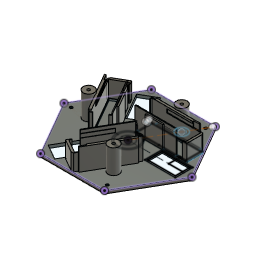
Inside Omniwheels 90D (Autodesk Fusion 360 archive; units mm, degrees)
design "Celluo V2.1 OmniWheels" references "Motor 90 shaft"
Autodesk Fusion 360 part; units mm, degrees
note: some values were not read from the file. Chosen so that the rebuilt part matches the saved one: a direction; a side; which face or edge a step refers to; which sketch regions a step uses.
imported_body "Derived Base Feature3" makes body 1
sketch "Sketch10" plane through (0, 0, 0) normal (0, 1, 0) x (1, 0, 0)
  circle A0 centre (0, 0) radius 46
  line L0 (46, 0) -> (23, 39.8372)
  line L1 (23, 39.8372) -> (-23, 39.8372)
  line L2 (-23, 39.8372) -> (-46, 0)
  line L3 (-46, 0) -> (-23, -39.8372)
  line L4 (-23, -39.8372) -> (23, -39.8372)
  line L5 (23, -39.8372) -> (46, 0)
  line L6 (-21.2679, 36.8372) -> (-42.5359, 0)
  line L7 (-42.5359, 0) -> (-21.2679, -36.8372)
  line L8 (-21.2679, -36.8372) -> (21.2679, -36.8372)
  line L9 (21.2679, -36.8372) -> (42.5359, 0)
  line L10 (42.5359, 0) -> (21.2679, 36.8372)
  line L11 (21.2679, 36.8372) -> (-21.2679, 36.8372)
  line L12 (-22.134, 38.3372) -> (-44.2679, 0)
  line L13 (-44.2679, 0) -> (-22.134, -38.3372)
  line L14 (-22.134, -38.3372) -> (22.134, -38.3372)
  line L15 (22.134, -38.3372) -> (44.2679, 0)
  line L16 (44.2679, 0) -> (22.134, 38.3372)
  line L17 (22.134, 38.3372) -> (-22.134, 38.3372)
  line L18 (-21.9608, 38.0372) -> (-43.9215, 0)
  line L19 (-43.9215, 0) -> (-21.9608, -38.0372)
  line L20 (-21.9608, -38.0372) -> (21.9608, -38.0372)
  line L21 (21.9608, -38.0372) -> (43.9215, 0)
  line L22 (43.9215, 0) -> (21.9608, 38.0372)
  line L23 (21.9608, 38.0372) -> (-21.9608, 38.0372)
  line L24 (0, 0) -> (23, 39.8372) construction
  circle A1 centre (19.5, 33.775) radius 3.5
  circle A2 centre (19.5, 33.775) radius 2.1
  dimension "d727" = 92
  dimension "d729" = -1.5
  dimension "d730" = -1.8
  dimension "d891" = 7
  dimension "d892" = 39
  dimension "d893" = 4.2
  constraint coincident A0.centre L24.start
  constraint coincident A0 L0.start
  constraint coincident L24 A1.centre
  constraint concentric A1 A2
  measures "d727" diameter of A0
  measures "d891" diameter of A1
  measures "d892" distance of A0.centre A1.centre
  measures "d893" diameter of A2
extrude "Extrude1" add sketch "Sketch10" along normal blind 2 separate body contours L6 L7 L8 L9 L10 L11 A1 | L11 A1 | L10 L11 A1 | L10 L11 A1 | L10 A1 | L18 L19 L20 L21 L22 L23 | A2 makes body 2
sketch "Sketch11" plane through (0, 2, 0) normal (0, 1, 0) x (-1, 0, 0)
  circle A0 centre (0, 0) radius 6.9
  circle A1 centre (0, 0) radius 4.1
  line L0 (0, 0) -> (-28, 0) construction
  line L1 (3.783, -17.05) -> (5.0997, -17.05)
  line L2 (0, 0) -> (-21.2679, -36.8372) construction
  circle A2 centre (-13.5, -23.3827) radius 3.75
  circle A3 centre (-13.5, -23.3827) radius 2.1
  circle A4 centre (0, 0) radius 7.9
  line L3 (5.0997, -19.25) -> (5.1031, -19.95)
  line L4 (-21.9608, -38.0372) -> (21.9608, -38.0372)
  line L5 (21.9608, -38.0372) -> (43.9215, 0)
  line L6 (43.9215, 0) -> (21.9608, 38.0372)
  line L7 (21.9608, 38.0372) -> (-21.9608, 38.0372)
  line L8 (-21.9608, 38.0372) -> (-43.9215, 0)
  line L9 (-43.9215, 0) -> (-21.9608, -38.0372)
  line L10 (-28, 0) -> (-28, -8)
  line L11 (-28, -8) -> (-13.5, -8)
  line L12 (-13.5, -8) -> (1.5, -8)
  line L13 (1.5, -8) -> (1.5, -18)
  line L14 (1.5, -18) -> (-31.5, -18)
  line L15 (-31.5, -18) -> (-31.5, -8)
  line L16 (-28, -8) -> (-31.5, -8)
  line L17 (-28, -7.7) -> (-31.8, -7.7)
  line L18 (-31.8, -18.3) -> (-31.8, -7.7)
  line L19 (1.8, -18.3) -> (-31.8, -18.3)
  line L20 (1.8, -7.7) -> (1.8, -18.3)
  line L21 (-13.5, -7.7) -> (1.8, -7.7)
  line L22 (-28, -7.7) -> (-13.5, -7.7)
  line L23 (-28, -7.1) -> (-32.4, -7.1)
  line L24 (-32.4, -18.9) -> (-32.4, -7.1)
  line L25 (2.4, -18.9) -> (-32.4, -18.9)
  line L26 (2.4, -7.1) -> (2.4, -18.9)
  line L27 (-13.5, -7.1) -> (2.4, -7.1)
  line L28 (-28, -7.1) -> (-13.5, -7.1)
  line L29 (-28, 0) -> (-37.5, 0)
  line L30 (-37.5, 0) -> (-37.5, -5)
  line L31 (-37.5, -5) -> (-18.5, -5)
  line L32 (-18.5, -5) -> (-18.5, 5)
  line L33 (-18.5, 5) -> (-37.5, 5)
  line L34 (-37.5, 5) -> (-37.5, 0)
  line L35 (0, -18.9) -> (0, -19.9)
  line L36 (0, -19.9) -> (-30, -19.9)
  line L37 (-30, -19.9) -> (-30, -18.9)
  line L38 (-33.3242, -17.5) -> (-33.3242, -7.1)
  line L39 (-33.3242, -7.1) -> (-32.4, -7.1)
  line L40 (2.4, -9.0599) -> (1.5, -9.0599)
  line L41 (2.4, -17.2552) -> (1.5, -17.2552)
  line L42 (-5.55, -7.1) -> (-5.55, -6.1)
  line L43 (-5.55, -6.1) -> (-26, -6.1)
  line L44 (-26, -6.1) -> (-26, -7.1)
  line L45 (-17.6828, -6.1) -> (-17.6828, -7.1)
  line L46 (-26, -7.1) -> (-26, -8)
  line L47 (-30.2, -7.1) -> (-30.2, -8)
  line L48 (-38.5, 0) -> (-38.5, -6)
  line L49 (-38.5, -6) -> (-17.5, -6)
  line L50 (-17.5, -6) -> (-17.5, 6)
  line L51 (-17.5, 6) -> (-38.5, 6)
  line L52 (-38.5, 6) -> (-38.5, 0)
  line L53 (-32.4, -18.9) -> (-33.3242, -17.5)
  dimension "d733" = 13.8
  dimension "d734" = 8.2
  dimension "d735" = 28
  dimension "d750" = 7.5
  dimension "d751" = 4.2
  dimension "d752" = 27
  dimension "d803" = 1
  dimension "d977" = 8
  dimension "d980" = 14.5
  dimension "d981" = 15
  dimension "d982" = 10
  dimension "d983" = 33
  dimension "d984" = 10
  dimension "d985" = -0.3
  dimension "d986" = -0.9
  dimension "d987" = 9.5
  dimension "d988" = 5
  dimension "d989" = 19
  dimension "d990" = 10
  dimension "d991" = 19
  dimension "d992" = 1
  dimension "d993" = 1
  dimension "d1000" = 1
  constraint coincident A0.centre A1.centre
  constraint concentric A0 A1
  constraint horizontal L0
  constraint coincident L2 A2.centre
  constraint concentric A2 A3
  constraint perpendicular L0 L10
  constraint perpendicular L10 L11
  constraint perpendicular L10 L12
  constraint perpendicular L13 L14
  constraint perpendicular L14 L15
  constraint perpendicular L15 L16
  constraint perpendicular L10 L29
  constraint perpendicular L29 L30
  constraint perpendicular L30 L31
  constraint perpendicular L31 L32
  constraint perpendicular L32 L33
  constraint coincident L25 L35.start
  constraint perpendicular L25 L35
  constraint perpendicular L35 L36
  constraint coincident L25 L37.end
  constraint perpendicular L25 L37
  constraint coincident L24 L23.end
  constraint perpendicular L24 L39
  constraint coincident L26 L40.start
  constraint coincident L13 L40.end
  constraint perpendicular L13 L40
  constraint coincident L26 L41.start
  constraint coincident L13 L41.end
  constraint perpendicular L13 L41
  constraint midpoint L27 L42.start
  constraint perpendicular L27 L42
  constraint perpendicular L42 L43
  constraint coincident L28 L44.end
  constraint perpendicular L28 L44
  constraint coincident L43 L45.start
  constraint coincident L28 L45.end
  constraint perpendicular L28 L45
  constraint coincident L11 L46.end
  constraint perpendicular L11 L46
  constraint midpoint L23 L47.start
  constraint coincident L16 L47.end
  constraint perpendicular L16 L47
  constraint vertical L38
  constraint collinear L23 L39
  measures "d733" diameter of A0
  measures "d734" diameter of A1
  measures "d735" distance of A0.centre L0.end
  measures "d750" diameter of A2
  measures "d751" diameter of A3
  measures "d752" distance of A0.centre A2.centre
  measures "d977" distance of L0.end L10.end
  measures "d980" distance of L10.end L11.end
  measures "d981" distance of L11.end L12.end
  measures "d982" distance of L12.end L13.end
  measures "d983" distance of L13.end L14.end
  measures "d984" distance of L14.end L15.end
  measures "d987" distance of L0.end L29.end
  measures "d988" distance of L29.end L30.end
  measures "d989" distance of L30.end L31.end
  measures "d990" distance of L31.end L32.end
  measures "d991" distance of L32.end L33.end
  measures "d992" distance of L35.start L35.end
  measures "d993" distance of L42.start L42.end
sketch "Sketch14" plane through (0, 2, 0) normal (0, 1, 0) x (-1, 0, 0)
  line L0 (0, 0) -> (-33, -19) construction
  line L1 (-3.5532, -2.0458) -> (-4.5485, -0.317)
  circle A0 centre (0, 0) radius 4.1
  line L2 (-44, 0) -> (-22, -38)
  line L3 (-21.9608, -38.0372) -> (21.9608, -38.0372)
  line L4 (21.9608, -38.0372) -> (43.9215, 0)
  line L5 (43.9215, 0) -> (21.9608, 38.0372)
  line L6 (21.9608, 38.0372) -> (-21.9608, 38.0372)
  line L7 (-21.9608, 38.0372) -> (-43.9215, 0)
  line L8 (-43.9215, 0) -> (-21.9608, -38.0372)
  constraint coincident L0.start A0.centre
  constraint coincident L0 L1.start
  constraint perpendicular L0 L1
  constraint tangent L1 A0
  constraint midpoint L0.end L2
ref_plane "WorkPlane3" through (4.0508, 2, -1.1814) normal (-0.750517, -0.5, 0.432116) x (0.498964, 0, 0.866622)
sketch "Sketch15" plane through (4.0508, 2, -1.1814) normal (-0.750517, -0.5, 0.432116) x (0.498964, 0, 0.866622)
  line L0 (-0.9974, 0) -> (-0.9974, 2)
  line L1 (-0.9974, 0) -> (-2.7974, 0)
  line L2 (-2.7974, 0) -> (-2.7974, 2)
  line L3 (-2.7974, 2) -> (-0.9974, 2)
  line L4 (-2.7974, 0) -> (-2.7974, -2)
  line L5 (-2.7974, -2) -> (-0.9977, -2)
  line L6 (-0.9977, -2) -> (-0.9974, 0)
  line L7 (0.8026, 0) -> (0.8026, 2)
  line L8 (0.8026, 2) -> (-0.9974, 2)
  line L9 (0.8026, 0) -> (0.8026, -2)
  line L10 (0.8026, -2) -> (-0.997, -2)
  line L11 (-0.997, -2) -> (-0.9974, 0)
  line L12 (-3.2974, -2.5) -> (-0.9977, -2.5)
  line L13 (-3.2974, 0) -> (-3.2974, -2.5)
  line L14 (-3.2974, 0) -> (-3.2974, 2.5)
  line L15 (-3.2974, 2.5) -> (-0.9974, 2.5)
  line L16 (1.3026, 2.5) -> (-0.9974, 2.5)
  line L17 (1.3026, 0) -> (1.3026, 2.5)
  line L18 (1.3026, 0) -> (1.3026, -2.5)
  line L19 (1.3026, -2.5) -> (-0.997, -2.5)
  line L20 (-0.997, -2.5) -> (-0.9977, -2.5)
  line L21 (-3.2974, -2) -> (1.3026, -2)
  point P0 (-0.9974, 0)
  dimension "d805" = 2
  dimension "d806" = 1.8
  dimension "d807" = 2
  dimension "d940" = 0.5
  constraint coincident P0 L0.start
  constraint perpendicular L0 L1
  constraint perpendicular L1 L2
  constraint perpendicular L1 L4
  constraint perpendicular L4 L5
  constraint symmetric P0 L0 L1.start
  constraint symmetric L3.end L0 L8.end
  constraint symmetric L0 L1.end L7.start
  constraint symmetric L0 L2.end L7.end
  constraint symmetric L0 L4.end L9.end
  constraint symmetric L0 L5.end L10.end
  constraint parallel L12 L20
  constraint coincident L13 L21.start
  constraint coincident L18 L21.end
  constraint perpendicular L18 L21
  measures "d805" distance of P0 L0.end
  measures "d806" distance of P0 L1.end
  measures "d807" distance of L1.end L4.end
extrude "Extrude9" add sketch "Sketch15" against normal blind 3 contours L0 L1 L2 L3 | L1 L4 L5 L6 L11 L21 | L0 L6 L7 L8 L9 L10 L11 L21 | L2 L3 L4 L7 L8 L9 L13 L14 L15 L16 L17 L18 L21 bodies 2
sketch "Sketch16" plane through (5.6669, 3.7754, -3.2628) normal (0.750517, 0.5, -0.432116) x (-0.498964, 0, -0.866622)
  line L0 (-2.3, -2.05) -> (2.3, -2.05)
  line L1 (0.95, -1.25) -> (-0.95, -1.25)
  line L2 (-0.95, -1.25) -> (-0.95, 1.25)
  line L3 (-0.95, 1.25) -> (0.95, 1.25)
  line L4 (0.95, 1.25) -> (0.95, -1.25)
  line L5 (0.95, -1.25) -> (-0.95, 1.25) construction
  line L6 (-0.95, -1.25) -> (0.95, 1.25) construction
  line L7 (2.3, -2.05) -> (2.3, 2.1821)
  line L8 (2.3, 2.1821) -> (-2.3, 2.1821)
  line L9 (-2.3, 2.1821) -> (-2.3, -2.05)
  dimension "d941" = 1.9
  dimension "d942" = 2.5
  constraint horizontal L1
  constraint perpendicular L1 L2
  constraint parallel L1 L3
  constraint parallel L2 L4
  constraint coincident L5 origin
  constraint coincident L6 origin
  measures "d941" distance of L2.end L3.end
  measures "d942" distance of L1.start L3.end
extrude "Extrude10" cut sketch "Sketch16" against normal blind 8.5 contours L1 L2 L3 L4 bodies 2
sketch "Sketch17" plane through (-0.9455, 1.8897, 0.5444) normal (-0.433311, 0.866025, 0.249482) x (0.498964, 0, 0.866622)
  line L0 (-1.8, 4.5507) -> (1.8, 4.5507)
  line L1 (1.8, 7.5507) -> (-1.8, 7.5507)
  line L2 (-1.8, 7.5507) -> (-1.8, 4.5507)
  line L3 (1.8, 4.5507) -> (1.8, 7.5507)
  line L4 (-1.8, 6.0507) -> (1.8, 6.0507) construction
  line L5 (0, 6.0507) -> (-1.5, 6.0507)
  line L6 (-1.5, 6.0507) -> (-1.5, 5.0507)
  line L7 (-1.5, 5.0507) -> (1.5, 5.0507)
  line L8 (1.5, 5.0507) -> (1.5, 7.0507)
  line L9 (1.5, 7.0507) -> (-1.5, 7.0507)
  line L10 (-1.5, 7.0507) -> (-1.5, 6.0507)
  line L11 (1.0425, 7.0507) -> (1.0425, 7.5803)
  line L12 (0, 6.0507) -> (0, 7.5507) construction
  line L13 (-1.0425, 7.0507) -> (-1.0425, 7.5803)
  line L14 (-1.0425, 7.5803) -> (1.0425, 7.5803)
  line L15 (-2.3, 4.5507) -> (2.3, 4.5507)
  line L16 (2.3, 4.5507) -> (2.3, 7.5507)
  line L17 (2.3, 7.5507) -> (-2.3, 7.5507)
  line L18 (-2.3, 7.5507) -> (-2.3, 4.5507)
  dimension "d814" = 1.5
  dimension "d815" = 1
  dimension "d816" = 3
  dimension "d817" = 2
  constraint midpoint L2 L4.start
  constraint midpoint L3 L4.end
  constraint parallel L4 L5
  constraint perpendicular L5 L6
  constraint perpendicular L6 L7
  constraint perpendicular L7 L8
  constraint horizontal L9
  constraint coincident L9 L11.start
  constraint vertical L11
  constraint midpoint L1 L12.end
  constraint perpendicular L1 L12
  constraint symmetric L11.start L12 L13.start
  constraint symmetric L11.end L12 L13.end
  measures "d814" distance of L5.start L5.end
  measures "d815" distance of L5.end L6.end
  measures "d816" distance of L6.end L7.end
  measures "d817" distance of L7.end L8.end
extrude "Extrude12" cut sketch "Sketch17" against normal blind 3.2 contours L1 L11 L13 L14 L17 | L1 L9 L11 L13 L17 | L6 L7 L8 L9 L10 bodies 2
pattern_circular "C-Pattern4" count 3 over 360 about axis through (0, 1.75, 0) along (0, 1, 0) of "Extrude9", "Extrude10", "Extrude12"
extrude "Extrude8" cut sketch "Sketch11" against normal up to surface (2 mm away) contours A1 bodies 2
extrude "Extrude5" add sketch "Sketch11" along normal blind 16.1 contours A2 L36 | A2 L36 | A4 L21 L26 L27 | A4 L21 L22 L27 L28 L46 | A3 bodies 2
extrude "Extrude6" add sketch "Sketch11" along normal blind 15 contours A2 L25 L35 L36 L37 | L17 L18 L19 L20 L23 L24 L25 L26 L41 L47 | L24 L38 L39 L53 | A4 L20 L21 L26 L40 | A4 L21 L26 L27 | A4 L21 L22 L27 L28 L46 | L27 L28 L42 L43 L45 bodies 2
sketch "Sketch22" plane through (0, 17, 0) normal (0, 1, 0) x (-1, 0, 0)
  line L0 (5.0997, -13) -> (3.883, -13)
  line L1 (5.0997, -11.5) -> (3.883, -11.5)
  line L2 (5.0997, -14.5) -> (3.883, -14.5)
  line L3 (1.7664, -7.7) -> (1.8, -7.7)
  line L4 (1.8, -7.7) -> (1.8, -9.0599)
  line L5 (1.8, -9.0599) -> (2.4, -9.0599)
  line L6 (2.4, -9.0599) -> (2.4, -7.5266)
  line L7 (-17.6828, -7.1) -> (-5.55, -7.1)
  line L8 (-5.55, -7.1) -> (-5.55, -6.1)
  line L9 (-5.55, -6.1) -> (-17.6828, -6.1)
  line L10 (-17.6828, -6.1) -> (-17.6828, -7.1)
  line L11 (-12.1095, -19.9) -> (0, -19.9)
  line L12 (0, -19.9) -> (0, -18.9)
  line L13 (0, -18.9) -> (2.4, -18.9)
  line L14 (2.4, -18.9) -> (2.4, -17.2552)
  line L15 (2.4, -17.2552) -> (1.8, -17.2552)
  line L16 (1.8, -17.2552) -> (1.8, -18.3)
  line L17 (1.8, -18.3) -> (-31.8, -18.3)
  line L18 (-31.8, -18.3) -> (-31.8, -7.7)
  line L19 (-31.8, -7.7) -> (-30.2, -7.7)
  line L20 (-30.2, -7.7) -> (-30.2, -7.1)
  line L21 (-30.2, -7.1) -> (-33.3242, -7.1)
  line L22 (-33.3242, -7.1) -> (-33.3242, -17.5)
  line L23 (-32.4, -18.9) -> (-30, -18.9)
  line L24 (-30, -18.9) -> (-30, -19.9)
  line L25 (-30, -19.9) -> (-14.8905, -19.9)
  arc A0 (1.7664, -7.7) -> (2.4, -7.5266) centre (0, 0) ccw
  arc A1 (-12.1095, -19.9) -> (-14.8905, -19.9) centre (-13.5, -23.3827) ccw
  line L26 (-33.3242, -17.5) -> (-32.4, -18.9)
  dimension "d943" = 1.5
  dimension "d944" = 1.5
  measures "d943" distance of L0 L2
  measures "d944" distance of L0 L1
extrude "Extrude7" add sketch "Sketch11" along normal blind 16.5 contours A2 L36 | A2 L36 | A3 bodies 2
sketch "Sketch19" plane through (33.3242, 0, 0) normal (1, 0, 0) x (0, 0, -1)
  line L0 (18.8186, 13.2) -> (18.8186, 15.7)
  line L1 (7.5, 13.2) -> (7.5, 15.7)
  line L2 (7.5, 15.7) -> (18.8186, 15.7)
  line L3 (18.8186, 13.2) -> (7.5, 13.2)
  line L4 (7.57, 15.63) -> (18.7486, 15.63)
  line L5 (18.7486, 13.27) -> (18.7486, 15.63)
  line L6 (18.7486, 13.27) -> (7.57, 13.27)
  line L7 (7.57, 13.27) -> (7.57, 15.63)
  line L8 (6.35, 2) -> (6.4273, 2)
  line L9 (7.3, 2) -> (9, 2)
  line L10 (7.3, 2) -> (7.3, 17)
  line L11 (7.6, 15.63) -> (7.6, 15.9409)
  line L12 (7.6, 15.9409) -> (18, 15.9409)
  line L13 (18, 15.9409) -> (18, 15.7)
  line L14 (0, 2) -> (38.0372, 2)
  line L15 (7.1, 2) -> (17.5, 2)
  line L16 (17.5, 2) -> (17.5, 17)
  line L17 (17.5, 17) -> (7.1, 17)
  line L18 (7.1, 17) -> (7.1, 2)
  line L19 (19.0186, 2) -> (19.0186, 17)
  line L20 (7.1, 13.2) -> (19.0186, 13.2)
  line L21 (19.0186, 13.2) -> (19.0186, 17)
  line L22 (19.0186, 17) -> (7.1, 17)
  dimension "d824" = 2.5
  dimension "d826" = 2.5
  dimension "d828" = -0.07
  dimension "d995" = 0.2
  dimension "d997" = 11.2
  dimension "d1010" = 0.2
  constraint perpendicular L0 L3
  constraint coincident L4 L11.start
  constraint perpendicular L4 L11
  constraint perpendicular L11 L12
  constraint coincident L2 L13.end
  constraint perpendicular L2 L13
  constraint midpoint L14 L19.start
  constraint perpendicular L14 L19
  constraint coincident L18 L20.start
  constraint coincident L19 L20.end
  constraint perpendicular L19 L20
  constraint coincident L17.end L18.start
  measures "d824" distance of L0.start L0.end
  measures "d826" distance of L1.start L1.end
  measures "d995" distance of L1 L10
  measures "d997" distance of L3 L14
  measures "d1010" distance of L0 L19
extrude "Extrude13" cut sketch "Sketch19" against normal blind 25 contours L0 L2 L3 L4 L5 L6 L16 L20 | L1 L2 L3 L4 L6 L7 L11 L16 L20 | L2 L12 L13 L16 | L4 L5 L6 L16 | L4 L6 L7 L16 | L2 L4 L11 L16 | L2 L11 L12 L16 bodies 2
extrude "Extrude22" cut sketch "Sketch19" against normal up to surface (7.3242 mm away) contours L0 L2 L3 L4 L5 L6 L16 L20 | L0 L2 L12 L13 L16 L19 L20 L21 L22 | L1 L2 L3 L4 L6 L7 L11 L16 L20 | L1 L2 L10 L11 L12 L16 L17 L20 L22 | L10 L17 L18 L20 L22 bodies 2
extrude "Extrude14" add sketch "Sketch19" against normal up to surface (24.9 mm away) separate body contours L4 L5 L6 L16 | L4 L6 L7 L16 makes body 3
hole "Hole1" at (13.5, 18.5, -23.3827) direction (0, -1, 0) diameter 1.85 depth 17.4 tip angle 118 bodies 2
extrude "Extrude19" cut sketch "Sketch11" against normal blind 1.2 contours L11 L12 L13 L14 L15 L16 bodies 2
extrude "Extrude20" cut sketch "Sketch11" against normal up to surface (2 mm away) contours L10 L29 L31 L32 L33 L34 | L10 L29 L30 L31 | L48 L49 L50 L51 L52 bodies 2
pattern_circular "C-Pattern5" count 3 over 360 about axis through (0, 1.75, 0) along (0, 1, 0) of "Extrude5", "Extrude6", "Extrude7", "Extrude13", "Extrude22", "Extrude14", "Hole1", "Extrude19", "Extrude20" makes body 4 makes body 5
extrude "Extrude21" cut sketch "Sketch10" along normal blind 0.4 contours A2 bodies 2
hole "Hole6" at (19.5, 0.4, -33.775) direction (0, 1, 0) diameter 2 depth 8 tip angle 118 countersink diameter 4 countersink angle 90 bodies 2
pattern_circular "C-Pattern6" count 3 over 360 about axis through (0, 1.75, 0) along (0, 1, 0) of "Extrude21", "Hole6"
other "ExternalDerived7"
move_body "Move1" bodies 1 to x (0, 1, 0) y (0, 0, 1) z (1, 0, 0) at (-18, 7, 29)
move_body "Move2" bodies 1 to x (1, 0, 0) y (0, 1, 0) z (0, 0, 1) at (16.5316, 0, -42.0606)
hidden bodies 3 4 5 1
equation "BaseDiameter = 92 mm"
equation "CameraHole = 8.2 mm"
equation "BallDiameter = 16 mm"
equation "PCBHeight = 16.5 mm"
equation "PCBDiamete = 60 mm"
equation "OutterWallThickness = 3 mm"
equation "InnerWallThickness = 1 mm"
equation "Tolerance = 0.2 mm"
equation "MotorLenght = 24.4 mm"
equation "MotorDiameter = 12.1 mm"
equation "MotorWidth = 10.1 mm"
equation "MotorShaft = 10 mm" comment "Shaft and preShaft. Shaft 9.3"
equation "MotorMagnetWidth = 5 mm"
equation "MotorMagnetDiameter = 10 mm"
equation "PilarDistance = 27 mm"
equation "PilarDiameter = 7.5 mm"
equation "ScrewPilarDiameter = ScrewDiameter"
equation "ScrewPilarLength = 8 mm"
equation "MotorShaftDiameter = 3 mm"
equation "ScrewLidDiameter = ScrewDiameter"
equation "ScrewLidDistance = BaseDiameter / 2 - OutterWallThickness - ScrewHead"
equation "TopDiameter = 82 mm"
equation "ModuleHeight = 32 mm" comment "Original 30"
equation "CylinderScrewDiameter = 7 mm"
equation "ScrewHead = 4 mm" comment "for m3 5.5 test okey"
equation "CameraHoleBig = 13.8 mm"
equation "DistanceBallToWall = 1 mm"
equation "BallCaseThickness = 2.3 mm"
equation "BallDistance = 28 mm"
equation "BallMiddlePlane = 4.5 mm" comment "Old 4"
equation "BaseThickness = 2 mm"
equation "BottomLidThickness = 1 mm"
equation "BottomLEDWidth = 2.95 mm"
equation "BottomLEDHeight = 3.15 mm"
equation "MotorHole = 0.5 mm"
equation "BearingDiameter = 3 mm"
equation "MotorCylinderLength = 15.3 mm"
equation "SpacerDiameter = 4 mm"
equation "SpacerHeight = 4 mm"
equation "ScrewBottomLidHeight = 8 mm"
equation "ScrewLidHeight = 8 mm"
equation "PogoDistanceCenter = 27.3 mm"
equation "PogoDiameter = 1.7 mm" comment "Old 1.6"
equation "PogoDistance = 2.54 mm"
equation "MagnetConnectDiameter = 4.85 mm"
equation "MagnetConnectDepth = 1.65 mm - 0.15 mm"
equation "MagnetConnectDistanceCenter = 18 mm"
equation "MechanicalLockDistanceCenter = 12 mm"
equation "MechanicalLockLength = 15 mm"
equation "MechanicalLockWidth = 2 mm"
equation "MechanicalLockDepth = 1.5 mm"
equation "MechanicalLockFillet = 1 mm"
equation "BordersSoftness = 0.1 mm"
equation "BorderRadius = 1.5 mm"
equation "LidBallReduction = 2.5 mm"
equation "TouchBandWidth = 10 mm"
equation "ScrewPreHole = 0.4 mm"
equation "ScrewDiameter = 1.85 mm" comment "M2 = 1.85, M3=2.85"
equation "CameraDiameter = 20 mm"
equation "Game = 0.17 mm"
equation "MotorBaseSupport = 0.5 mm"
equation "d727 = BaseDiameter"
equation "d728 = -OutterWallThickness"
equation "d731 = BaseThickness"
equation "d733 = CameraHoleBig"
equation "d734 = CameraHole"
equation "d735 = BallDistance"
equation "MotorPreShaft = 0.7 mm"
equation "d752 = PilarDistance"
equation "d795 = MotorDiameter + 4 mm"
equation "d799 = PCBHeight"
equation "d834 = ScrewDiameter"
equation "d891 = CylinderScrewDiameter"
equation "d892 = ScrewLidDistance"
equation "d893 = ScrewHead + Tolerance"
equation "d1003 = ScrewPreHole"
equation "d1008 = ScrewHead"
equation "d865 = ScrewPreHole"
equation "d878 = ScrewDiameter"
equation "d880 = ScrewHead"
equation "d883 = ScrewDiameter"
equation "d885 = ScrewHead"
equation "d897 = ScrewDiameter"
equation "d899 = 4.00 mm - 0.5 mm"
equation "d902 = ScrewDiameter"
equation "d904 = 4.00 mm - 0.5 mm"
named bodies: "Base", "MotorLid", "MotorLid (1)", "MotorLid (2)", "Body1"

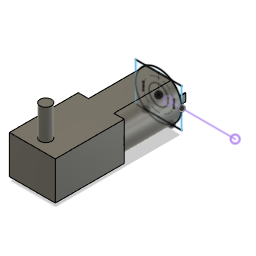
design "Motor 90 shaft"
Autodesk Fusion 360 part; units mm, degrees
sketch "Sketch1" plane through (0, 0, 0) normal (0, 0, 1) x (1, 0, 0)
  circle A0 centre (0, 0) radius 6
  line L0 (0, 0) -> (0, 5) construction
  line L1 (0, 5) -> (3.3166, 5)
  line L2 (0, 5) -> (-3.3166, 5)
  line L3 (20, 0) -> (2.5, 0)
  line L4 (0, -5) -> (3.3166, -5)
  line L5 (0, -5) -> (-3.3166, -5)
  circle A1 centre (0, 0) radius 2.5
  circle A2 centre (0, 0) radius 3.9 construction
  line L6 (-3.9, 0) -> (-3.9, 1)
  line L7 (-3.9, 1) -> (-4.1, 1)
  line L8 (-4.1, 1) -> (-4.1, -1)
  line L9 (-4.1, -1) -> (-3.9, -1)
  line L10 (-3.9, -1) -> (-3.9, 0)
  line L11 (4.1, 1) -> (4.1, -1)
  line L12 (3.9, 0) -> (3.9, 1)
  line L13 (3.9, 1) -> (4.1, 1)
  line L14 (3.9, -1) -> (3.9, 0)
  line L15 (4.1, -1) -> (3.9, -1)
  line L16 (6, 0) -> (6, 5)
  line L17 (6, 5) -> (-6, 5)
  line L18 (-6, 5) -> (-6, -5)
  line L19 (-6, -5) -> (6, -5)
  line L20 (6, -5) -> (6, 0)
  dimension "d1" = 12
  dimension "d2" = 5
  dimension "d5" = 5
  dimension "d8" = 7.8
  dimension "d9" = 1
  dimension "d10" = 0.2
  dimension "d11" = 2
  dimension "d12" = 0.2
  dimension "d15" = 5
  dimension "d16" = 12
  dimension "d17" = 10
  dimension "d18" = 12
  constraint coincident A0.centre L0.start
  constraint vertical L0
  constraint coincident A0 L1.end
  constraint perpendicular L0 L1
  constraint coincident A0 L2.end
  constraint perpendicular L0 L2
  constraint symmetric L0.end L3 L4.start
  constraint symmetric L1.end L3 L4.end
  constraint symmetric L2.end L3 L5.end
  constraint concentric A1 A2
  constraint coincident A2 L6.start
  constraint tangent A2 L6
  constraint vertical L6
  constraint perpendicular L6 L7
  constraint perpendicular L7 L8
  constraint perpendicular L8 L9
  constraint symmetric L0 L6.start L12.start
  constraint symmetric L0 L6.end L12.end
  constraint symmetric L0 L7.end L11.start
  constraint symmetric L0 L8.end L11.end
  constraint symmetric L0 L9.end L14.start
  constraint coincident L3 L16.start
  constraint perpendicular L3 L16
  constraint perpendicular L16 L17
  constraint perpendicular L2 L18
  constraint perpendicular L18 L19
  measures "d1" diameter of A0
  measures "d2" distance of A0.centre L0.end
  measures "d5" diameter of A1
  measures "d8" diameter of A2
  measures "d9" distance of L6.start L6.end
  measures "d10" distance of L6.end L7.end
  measures "d11" distance of L7.end L8.end
  measures "d12" distance of L8.end L9.end
  measures "d15" distance of L16.start L16.end
  measures "d16" distance of L16.end L17.end
  measures "d17" distance of L17.end L18.end
  measures "d18" distance of L18.end L19.end
extrude "Extrude1" add sketch "Sketch1" along normal blind 15 contours A0 L1 L2 L4 L5 L17 L19 | L3 L11 L14 L15 | L3 L11 L12 L13 | A1 | L6 L7 L8 L9 L10
extrude "Extrude2" add sketch "Sketch1" against normal blind 1.7 contours A1
extrude "Extrude3" add sketch "Sketch1" against normal blind 3 contours L3 L11 L14 L15 | L3 L11 L12 L13 | L6 L7 L8 L9 L10
extrude "Extrude4" add sketch "Sketch1" along normal blind 18 from surface at 15 contours A0 L1 L2 L4 L5 L17 L19 | A0 L19 L20 | A0 L16 L17 | A0 L17 L18 | A0 L18 L19 | L3 L11 L14 L15 | L3 L11 L12 L13 | A1 | L6 L7 L8 L9 L10
sketch "Sketch2" plane through (0, 5, 0) normal (0, 1, 0) x (-1, 0, 0)
  line L0 (-15, 0) -> (-15, 5)
  line L1 (-15, 5) -> (-33, 5)
  line L2 (-33, 5) -> (-33, -5)
  line L3 (-33, -5) -> (-15, -5)
  line L4 (-15, -5) -> (-15, 0)
  line L5 (-15, 0) -> (-31, 0) construction
  line L6 (-31, 0) -> (-29.5, 0) construction
  circle A0 centre (-29.5, 0) radius 1.5
  line L7 (-3.3166, 0) -> (3.3166, 0)
  line L8 (3.3166, 0) -> (3.3166, 15)
  line L9 (3.3166, 15) -> (6, 15)
  line L10 (6, 15) -> (6, 33)
  line L11 (6, 33) -> (-6, 33)
  line L12 (-6, 33) -> (-6, 15)
  line L13 (-6, 15) -> (-3.3166, 15)
  line L14 (-3.3166, 15) -> (-3.3166, 0)
  line L15 (3.3166, 15) -> (-3.3166, 15)
  line L16 (0, 15) -> (0, 31) construction
  line L17 (0, 31) -> (0, 29.5) construction
  circle A1 centre (0, 29.5) radius 1.5
  dimension "d22" = 16
  dimension "d23" = 1.5
  dimension "d24" = 3
  dimension "d25" = 16
  dimension "d26" = 1.5
  dimension "d27" = 3
  constraint coincident L0.start L4.end
  constraint perpendicular L0 L5
  constraint parallel L5 L6
  constraint coincident L6.end A0.centre
  constraint coincident L8.end L9.start
  constraint coincident L13.end L14.start
  constraint midpoint L15 L16.start
  constraint perpendicular L15 L16
  constraint parallel L16 L17
  constraint coincident L17.end A1.centre
  measures "d22" distance of L0.start L5.end
  measures "d23" distance of L5.end L6.end
  measures "d24" diameter of A0
  measures "d25" distance of L16.start L16.end
  measures "d26" distance of L16.end L17.end
  measures "d27" diameter of A1
extrude "Extrude5" add sketch "Sketch2" along normal blind 8 contours A1
